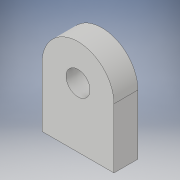
# Autodesk Inventor part: SUJECION_BALSA_UNDIMOTRIZ
Saved by Autodesk Inventor 2019.4 (Build 234330000, 330)
## iProperties
Created: 2020-08-20
Part Number: SUJECION_BALSA_UNDIMOTRIZ
Material: Generic
Document SubType Name: Modeling
Designer: crist
Density: 1 g/cm^3
Appearance: Default
Author: crist
Autodesk Inventor part; units mm, degrees
ref_plane "YZ Plane" through (0, 0, 0) normal (1, 0, 0) x (0, 1, 0)
ref_plane "XZ Plane" through (0, 0, 0) normal (0, 1, 0) x (-1, 0, 0)
ref_plane "XY Plane" through (0, 0, 0) normal (0, 0, 1) x (1, 0, 0)
sketch "Boceto1" plane through (0, 0, 0) normal (0, 0, 1) x (1, 0, 0)
  circle A0 centre (0, 0) radius 50
  circle A1 centre (0, 0) radius 150
  line L0 (150, -250) -> (150, 0)
  line L1 (150, -250) -> (-150, -250)
  line L2 (-150, -250) -> (-150, 0)
  dimension "d0" = 100
  dimension "d1" = 300
  dimension "d4" = 300
  constraints: 6 end point, 2 centre point, 2 coincident, 2 point on circle, 2 tangent, 1 horizontal
  measures "d0" diameter of A0
  measures "d1" diameter of A1
  measures "d4" distance of L0.start L1.end
extrude "Extrusión1" add sketch "Boceto1" along normal blind 100
